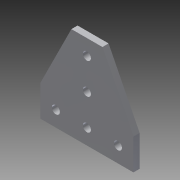
# Autodesk Inventor part: T joining plate
Saved by Autodesk Inventor 2014 SP1 (Build 180222100, 222)
## iProperties
Created: 2016-04-12
Part Number: T joining plate
Material: Generic
Document SubType Name: Modeling
Designer: Ben
Density: 1 g/cm^3
Appearance: Default
Author: Ben
Autodesk Inventor part; units mm, degrees
ref_plane "YZ Plane" through (0, 0, 0) normal (1, 0, 0) x (0, 1, 0)
ref_plane "XZ Plane" through (0, 0, 0) normal (0, 1, 0) x (-1, 0, 0)
ref_plane "XY Plane" through (0, 0, 0) normal (0, 0, 1) x (1, 0, 0)
sketch "Sketch1" plane through (0, 0, 0) normal (0, 0, 1) x (1, 0, 0)
  line L0 (30, -10) -> (-30, -10)
  line L1 (0, 30.1987) -> (0, -10) construction
  line L2 (-30, -10) -> (-30, 10)
  line L3 (-30, 10) -> (-10, 50)
  line L4 (-10, 50) -> (10, 50)
  line L5 (10, 50) -> (30, 10)
  line L6 (30, 10) -> (30, -10)
  circle A0 centre (0, 0) radius 2.6
  circle A1 centre (-20, 0) radius 2.6
  circle A2 centre (20, 0) radius 2.6
  circle A3 centre (0, 0) radius 2.6
  circle A4 centre (0, 20) radius 2.6
  circle A5 centre (0, 40) radius 2.6
  point P0 (0, 50)
  dimension "d2" = 20
  dimension "d3" = 20
  dimension "d4" = 60
  dimension "d5" = 60
  dimension "d6" = 5.2
  dimension "d8" = 10
  dimension "d11" = 20
  dimension "d14" = 20
  dimension "d19" = 20
  constraints: 14 end point, 6 centre point, 3 parallel, 2 horizontal, 2 midpoint, 2 point on line, 1 perpendicular, 1 vertical, 10 other
  measures "d2" distance of L0.end L2.end
  measures "d3" distance of L3.end L4.end
  measures "d4" distance between parallel lines of L0 L4
  measures "d5" distance of L0.start L0.end
  measures "d6" diameter of A0
  measures "d8" distance from line of L0 A0.centre
  measures "d11" distance of A0.centre A1.centre
  measures "d14" distance of A0.centre A2.centre
  measures "d19" distance of A0.centre A4.centre
extrude "Extrusion1" add sketch "Sketch1" along normal blind 4
body "Solid1"
